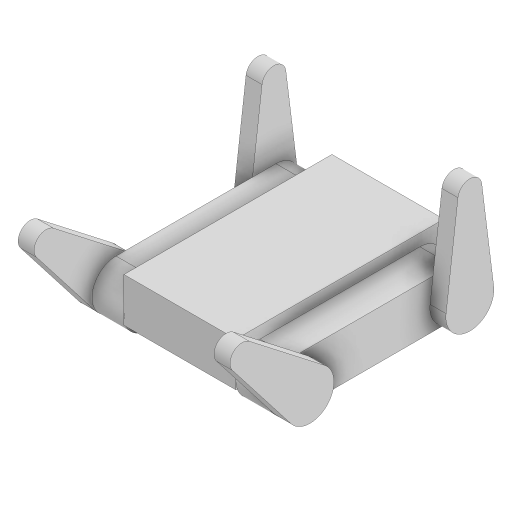
# Autodesk Inventor part: Dimensions(Roughly)
Saved by Autodesk Inventor 2023 (Build 270158030, 158C)
## iProperties
Created: 2022-09-21
Part Number: Dimensions(Roughly)
Material: Generic
Document SubType Name: Modeling
Designer: kumpu
Density: 1 g/cm^3
Appearance: Default
Author: kumpu
Autodesk Inventor part; units mm, degrees
ref_plane "YZ Plane" through (0, 0, 0) normal (1, 0, 0) x (0, 1, 0)
ref_plane "XZ Plane" through (0, 0, 0) normal (0, 1, 0) x (-1, 0, 0)
ref_plane "XY Plane" through (0, 0, 0) normal (0, 0, 1) x (1, 0, 0)
sketch "Sketch1" plane through (0, 0, 0) normal (0, 1, 0) x (-1, 0, 0)
  line L0 (-177.8, 330.2) -> (177.8, 330.2)
  line L1 (177.8, 330.2) -> (177.8, -330.2)
  line L2 (177.8, -330.2) -> (-177.8, -330.2)
  line L3 (-177.8, -330.2) -> (-177.8, 330.2)
  line L4 (-177.8, 330.2) -> (177.8, -330.2) construction
  line L5 (177.8, 330.2) -> (-177.8, -330.2) construction
  point P0 (0, 0)
  dimension "d0" = 355.6
  dimension "d1" = 660.4
  constraints: 12 end point, 2 midpoint, 2 parallel, 1 horizontal, 1 perpendicular
  measures "d0" distance of L0.start L0.end
  measures "d1" distance of L0.end L1.end
extrude "Extrusion1" add sketch "Sketch1" along normal blind 114.3 and the other way blind 25.4
sketch "Sketch2" plane through (177.8, -25.4, -330.2) normal (1, 0, 0) x (0, 0, -1)
  line L0 (-584.2, 25.4) -> (-76.2, 25.4) construction
  line L1 (-584.2, -50.8) -> (-76.2, -50.8)
  line L2 (-76.2, 101.6) -> (-584.2, 101.6)
  arc A0 (-584.2, 101.6) -> (-584.2, -50.8) centre (-584.2, 25.4) ccw
  arc A1 (-76.2, -50.8) -> (-76.2, 101.6) centre (-76.2, 25.4) ccw
  line L3 (-330.2, 25.4) -> (177.8, 25.4) construction
  line L4 (-330.2, 25.4) -> (-330.2, 0) construction
  line L5 (-660.4, 0) -> (0, 0) construction
  point P0 (-330.2, 25.4)
  dimension "d6" = 254
  dimension "d7" = 0
  dimension "d8" = 152.4
  dimension "d9" = 25.4
  constraints: 12 end point, 4 point on circle, 4 tangent, 2 centre point, 2 horizontal, 2 midpoint, 1 collinear, 1 parallel, 1 perpendicular
  measures "d6" distance of L3.start L0.end
  measures "d7" distance between parallel lines of L0 L3
  measures "d8" diameter of A1
  measures "d9" distance of L3.start L4.end
extrude "Extrusion2" add sketch "Sketch2" along normal blind 101.6
sketch "Sketch3" plane through (279.4, -25.4, -330.2) normal (1, 0, 0) x (0, 0, -1)
  circle A0 centre (-584.2, 25.4) radius 63.5
  circle A1 centre (-76.2, 25.4) radius 63.5
  arc A2 (-584.2, 101.6) -> (-584.2, -50.8) centre (-584.2, 25.4) ccw construction
  arc A3 (-76.2, -50.8) -> (-76.2, 101.6) centre (-76.2, 25.4) ccw construction
  point P0 (-330.2, 25.4)
  dimension "d12" = 127
  constraints: 2 centre point, 2 concentric, 1 equal radius
  measures "d12" diameter of A0
extrude "Extrusion3" add sketch "Sketch3" along normal blind 6.35
sketch "Sketch4" plane through (285.75, 0, 254) normal (1, 0, 0) x (0, 0, -1)
  line L0 (0, 0) -> (-215.5261, 215.5261) construction
  line L1 (46.7237, 60.1941) -> (-192.1643, 245.6232)
  line L2 (-245.6232, 192.1643) -> (-60.1941, -46.7237)
  arc A0 (-60.1941, -46.7237) -> (46.7237, 60.1941) centre (0, 0) ccw
  arc A1 (-192.1643, 245.6232) -> (-245.6232, 192.1643) centre (-215.5261, 215.5261) ccw
  arc A2 (0, 76.2) -> (0, -76.2) centre (0, 0) ccw construction
  line L3 (0, 0) -> (-144.2559, 0) construction
  line L4 (508, 0) -> (508, 304.8) construction
  line L5 (583.6023, 9.525) -> (545.8012, 309.5625)
  line L6 (470.1988, 309.5625) -> (432.3977, 9.525)
  arc A3 (432.3977, 9.525) -> (583.6023, 9.525) centre (508, 0) ccw
  arc A4 (545.8012, 309.5625) -> (470.1988, 309.5625) centre (508, 304.8) ccw
  circle A5 centre (508, 0) radius 63.5 construction
  point P0 (254, 0)
  point P1 (-107.7631, 107.7631)
  point P2 (508, 152.4)
  dimension "d15" = 304.8
  dimension "d17" = 38.1
  dimension "d20" = 45
  constraints: 18 end point, 8 point on circle, 8 tangent, 4 centre point, 3 equal radius, 2 concentric, 2 midpoint, 1 equal length, 1 horizontal, 1 vertical, 1 other
  measures "d15" distance of L0.start L0.end
  measures "d17" radius of A1
  measures "d20" angle of L0 L3
extrude "Extrusion4" add sketch "Sketch4" along normal blind 50.8
mirror "Mirror1" about plane through (0, 0, 0) normal (1, 0, 0) of "Extrusion2", "Extrusion4", "Extrusion3"
body "Solid1"
